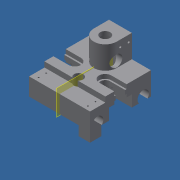
# Autodesk Inventor part: HotendMountCarriage
Saved by Autodesk Inventor 2021 (Build 250183000, 183)
## iProperties
Created: 2022-08-30
Part Number: HotendMountCarriage
Material: Generic
Document SubType Name: Modeling
Designer: Nathann
Density: 1 g/cm^3
Appearance: Default
Author: Nathann
Autodesk Inventor part; units mm, degrees
ref_plane "YZ Plane" through (0, 0, 0) normal (1, 0, 0) x (0, 1, 0)
ref_plane "XZ Plane" through (0, 0, 0) normal (0, 1, 0) x (-1, 0, 0)
ref_plane "XY Plane" through (0, 0, 0) normal (0, 0, 1) x (1, 0, 0)
sketch "Sketch1" plane through (0, 0, 0) normal (0, 0, 1) x (1, 0, 0)
  line L0 (0, 0) -> (80, 0)
  line L1 (80, 0) -> (80, -80)
  line L2 (80, -80) -> (0, -80)
  line L3 (0, -80) -> (0, 0)
  dimension "d0" = 80
  dimension "d1" = 80
  constraints: 8 end point, 2 parallel, 1 horizontal, 1 perpendicular
  measures "d0" distance of L0.start L0.end
  measures "d1" distance of L2.end L0.start
extrude "Extrusion1" add sketch "Sketch1" along normal blind 15
sketch "Sketch2" plane through (0, 0, 0) normal (0, 0, -1) x (-1, 0, 0)
  line L0 (0, 0) -> (-80, 0) projected
  circle A0 centre (-60, -40) radius 6.1
  line L1 (-80, 0) -> (-80, -80) projected
  line L2 (-60, -33.9) -> (-80, -33.9)
  line L3 (-80, -80) -> (-80, 0) projected
  line L4 (-60, -46.1) -> (-80, -46.1)
  line L5 (-80, -46.1) -> (-80, -33.9)
  dimension "d7" = 40
  dimension "d8" = 20
  dimension "d9" = 12.2
  constraints: 6 end point, 2 perpendicular, 2 point on circle, 2 point on line, 1 centre point, 1 horizontal
  measures "d7" distance from line of L0 A0.centre
  measures "d8" distance from line of L1 A0.centre
  measures "d9" diameter of A0
extrude "Extrusion2" cut sketch "Sketch2" against normal through all
sketch "Sketch3" plane through (0, 0, 0) normal (0, 0, -1) x (-1, 0, 0)
  arc A0 (-60, -46.1) -> (-60, -33.9) centre (-60, -40) ccw projected
  circle A1 centre (-60, -40) radius 8.1
  line L0 (-60, -31.9) -> (-80, -31.9)
  line L1 (-80, -33.9) -> (-80, 0) projected
  line L2 (-60, -48.1) -> (-80, -48.1)
  line L3 (-80, -48.1) -> (-80, -31.9)
  point P0 (0, 0)
  dimension "d12" = 16.2
  constraints: 6 end point, 2 horizontal, 2 point on circle, 1 centre point, 1 coincident, 1 perpendicular, 1 point on line
  measures "d12" diameter of A1
extrude "Extrusion3" cut sketch "Sketch3" against normal blind 4
sketch "Sketch4" plane through (0, 0, 15) normal (0, 0, 1) x (1, 0, 0)
  line L0 (80, -31.9) -> (60, -31.9) projected
  arc A0 (60, -31.9) -> (60, -48.1) centre (60, -40) ccw projected
  line L1 (60, -48.1) -> (80, -48.1) projected
  line L2 (80, -46.1) -> (60, -46.1) projected
  arc A1 (60, -33.9) -> (60, -46.1) centre (60, -40) ccw projected
  line L3 (60, -33.9) -> (80, -33.9) projected
  line L4 (80, -33.9) -> (80, -31.9)
  line L5 (80, -33.9) -> (80, 0) projected
  line L6 (80, -46.1) -> (80, -48.1)
  line L7 (80, -80) -> (80, -46.1) projected
  point P0 (0, 0)
  constraints: 4 end point, 2 collinear
extrude "Extrusion4" cut sketch "Sketch4" against normal blind 5.5
sketch "Sketch5" plane through (0, 0, 0) normal (0, 0, -1) x (-1, 0, 0)
  arc A0 (-60, -46.1) -> (-60, -33.9) centre (-60, -40) ccw projected
  line L0 (-80, -31.9) -> (-60, -31.9) projected
  circle A1 centre (-60, -40) radius 8.1
  line L1 (-60, -31.9) -> (-60, -31.9)
  line L2 (-73.8, -31.9) -> (-73.8, -48.1)
  line L3 (-60, -48.1) -> (-60, -48.1)
  arc A2 (-60, -48.1) -> (-60, -31.9) centre (-60, -40) ccw projected
  line L4 (-60, -31.9) -> (-60, -31.9)
  line L5 (-60, -31.9) -> (-60, -31.9)
  line L6 (-60, -33.9) -> (-60, -46.1)
  arc A3 (-60, -31.9) -> (-73.8, -31.9) centre (-66.9, -31.9) ccw
  arc A4 (-73.8, -48.1) -> (-60, -48.1) centre (-66.9, -48.1) ccw
  point P0 (0, 0)
  dimension "d17" = 13.8
  dimension "d20" = 16.2
  dimension "d21" = 8.1
  dimension "d37" = 0
  constraints: 8 end point, 7 point on circle, 4 tangent, 3 centre point, 3 vertical, 1 coincident, 1 parallel, 6 other
  measures "d17" distance of L1.end L2.start
  measures "d20" distance of A4.centre A3.centre
  measures "d21" vertical distance of A1.centre A3.centre
  measures "d37" distance of L0.end L1.end
extrude "Extrusion5" cut sketch "Sketch5" against normal blind 4 contours A3 L0 | L0 A1 A4 L2
sketch "Sketch6" plane through (80, 0, 15) normal (1, 0, 0) x (0, 0, -1)
  line L0 (15, 0) -> (0, 0) projected
  line L1 (15, 0) -> (30, 0)
  line L2 (30, -25) -> (15, -25)
  line L3 (15, -25) -> (15, 0)
  line L4 (15, -80) -> (0, -80) projected
  line L5 (15, -80) -> (30, -80)
  line L6 (30, -55) -> (15, -55)
  line L7 (15, -55) -> (15, -80)
  arc A0 (30, -4.4098) -> (30, -15.5902) centre (25, -10) ccw
  arc A1 (30, -64.4098) -> (30, -75.5902) centre (25, -70) ccw
  line L8 (30, 0) -> (30, -4.4098)
  line L9 (30, -15.5902) -> (30, -25)
  line L10 (30, -80) -> (30, -75.5902)
  line L11 (30, -64.4098) -> (30, -55)
  dimension "d22" = 25
  dimension "d23" = 25
  dimension "d24" = 15
  dimension "d25" = 15
  dimension "d29" = 15
  dimension "d32" = 15
  dimension "d33" = 5
  dimension "d34" = 5
  dimension "d38" = 15
  dimension "d39" = 15
  dimension "d40" = 60
  dimension "d41" = 10
  dimension "d42" = 10
  constraints: 20 end point, 6 parallel, 4 perpendicular, 4 point on circle, 2 centre point, 2 horizontal
  measures "d22" distance of L1.end L2.start
  measures "d23" distance of L5.end L6.start
  measures "d24" distance of L4.start L5.end
  measures "d25" distance of L0.start L1.end
  measures "d29" diameter of A0
  measures "d32" diameter of A1
  measures "d33" distance from line of L8 A0.centre
  measures "d34" distance from line of A1.centre L11
  measures "d38" distance of L2.start L2.end
  measures "d39" distance of L6.start L6.end
  measures "d40" distance of A0.centre A1.centre
  measures "d41" distance from line of L5 A1.centre
  measures "d42" distance from line of L1 A0.centre
extrude "Extrusion6" add sketch "Sketch6" against normal blind 80
ref_plane "Work Plane1" through (40, -33.9, 4) normal (1, 0, 0) x (0, 0, -1)
mirror "Mirror1" about plane through (40, -33.9, 4) normal (1, 0, 0) of "Extrusion5", "Extrusion4", "Extrusion3", "Extrusion2"
sketch "Sketch8" plane through (80, -48.1, 4) normal (1, 0, 0) x (0, 0, -1)
  line L0 (-11, 0) -> (-11, -31.9) projected
  line L1 (-11, -31.9) -> (-4, -31.9)
  line L2 (-4, -31.9) -> (-4, -11.7)
  line L3 (-4, -11.7) -> (-11, -11.7)
  line L4 (-11, -11.7) -> (-11, -31.9)
  point P0 (4, 48.1)
  dimension "d49" = 20.2
  dimension "d50" = 7
  constraints: 8 end point, 2 parallel, 1 horizontal, 1 perpendicular
  measures "d49" distance of L1.end L2.end
  measures "d50" distance of L2.end L3.end
extrude "Extrusion8" cut sketch "Sketch8" along normal through all both and the other way through all
sketch "Sketch9" plane through (80, -80, 8) normal (0, 0, 1) x (1, 0, 0)
  circle A0 centre (-7.6, 14.9) radius 0.95
  circle A1 centre (-7.6, 4.9) radius 0.95
  line L0 (0, 20.2) -> (0, 0) projected
  line L1 (0, 0) -> (-80, 0) projected
  point P0 (-80, 80)
  dimension "d53" = 1.9
  dimension "d54" = 1.9
  dimension "d55" = 7.6
  dimension "d56" = 7.6
  dimension "d57" = 10
  dimension "d58" = 4.9
  constraints: 2 centre point
  measures "d53" diameter of A0
  measures "d54" diameter of A1
  measures "d55" distance from line of A0.centre L0
  measures "d56" distance from line of A1.centre L0
  measures "d57" distance of A1.centre A0.centre
  measures "d58" distance from line of L1 A1.centre
extrude "Extrusion9" cut sketch "Sketch9" against normal blind 10
ref_plane "Work Plane2" through (40, -48.1, 4) normal (1, 0, 0) x (0, 0, -1)
mirror "Mirror2" about plane through (40, -48.1, 4) normal (1, 0, 0) of "Extrusion9"
sketch "Sketch10" plane through (0, 0, 15) normal (0, 0, 1) x (1, 0, 0)
  line L0 (80, -55) -> (0, -55) projected
  circle A0 centre (40, -55) radius 6
  point P0 (0, 0)
  dimension "d61" = 12
  constraints: 1 centre point, 1 midpoint
  measures "d61" diameter of A0
extrude "Extrusion10" cut sketch "Sketch10" against normal through all
sketch "Sketch11" plane through (0, 0, 15) normal (0, 0, 1) x (1, 0, 0)
  circle A0 centre (40, -20) radius 15
  circle A1 centre (40, -20) radius 10
  line L0 (80, -31.9) -> (80, 0) projected
  line L1 (80, 0) -> (0, 0) projected
  line L2 (55, -20) -> (55, -5)
  line L3 (80, -4.4098) -> (0, -4.4098) projected
  line L4 (55, -5) -> (40, -5)
  line L5 (40, -5) -> (25, -5)
  line L6 (25, -5) -> (25, -20)
  line L7 (55, -5) -> (25, -5)
  line L8 (25, -5) -> (25, 0)
  line L9 (25, 0) -> (55, 0)
  line L10 (55, 0) -> (55, -5)
  dimension "d64" = 30
  dimension "d65" = 20
  dimension "d66" = 40
  dimension "d67" = 20
  constraints: 16 end point, 4 perpendicular, 3 point on circle, 2 centre point, 2 parallel, 2 point on line, 1 coincident, 1 horizontal, 1 tangent
  measures "d64" diameter of A0
  measures "d65" diameter of A1
  measures "d66" distance from line of L0 A0.centre
  measures "d67" distance from line of L1 A0.centre
extrude "Extrusion11" add sketch "Sketch11" along normal blind 30 contours A0 | A0 L4 L2 | L5 L8 L3 L10 L4 | A0 L6 L5 | L3 L8 L1 L10
sketch "Sketch12" plane through (0, 0, 45) normal (0, 0, 1) x (1, 0, 0)
  circle A0 centre (40, -20) radius 10 projected
  circle A1 centre (40, -20) radius 6.5
  point P0 (0, 0)
  dimension "d70" = 13
  constraints: 1 centre point, 1 coincident
  measures "d70" diameter of A1
extrude "Extrusion12" add sketch "Sketch12" against normal blind 5
sketch "Sketch13" plane through (0, 0, 15) normal (0, 0, 1) x (1, 0, 0)
  circle A0 centre (40, -20) radius 6.5 projected
  circle A1 centre (40, -20) radius 10
  point P0 (0, 0)
  constraints: 1 centre point, 1 coincident
extrude "Extrusion13" cut sketch "Sketch13" against normal blind 35 contours A0 | A1
sketch "Sketch14" plane through (55, -20, 15) normal (1, 0, 0) x (0, 0, -1)
  circle A0 centre (-21.5, 5) radius 1.45
  circle A1 centre (-21.5, 16) radius 1.45
  line L0 (0, 20) -> (-30, 20) projected
  line L1 (-30, 0) -> (-30, 20) projected
  point P0 (15, 20)
  dimension "d75" = 2.9
  dimension "d76" = 2.9
  dimension "d77" = 11
  dimension "d78" = 4
  dimension "d79" = 8.5
  dimension "d80" = 8.5
  constraints: 2 centre point
  measures "d75" diameter of A0
  measures "d76" diameter of A1
  measures "d77" distance of A1.centre A0.centre
  measures "d78" distance from line of L0 A1.centre
  measures "d79" distance from line of A1.centre L1
  measures "d80" distance from line of A0.centre L1
extrude "Extrusion14" cut sketch "Sketch14" against normal blind 15
sketch "Sketch15" plane through (55, -20, 15) normal (1, 0, 0) x (0, 0, -1)
  circle A0 centre (-8, 0) radius 7.5
  line L0 (15, -10) -> (-25, -10) projected
  line L1 (4, -6) -> (-11, -6)
  line L2 (4, 6) -> (-11, 6)
  line L3 (0, -11.9) -> (0, 20) projected
  point P0 (15, 20)
  dimension "d83" = 6
  dimension "d84" = 15
  dimension "d85" = 8
  constraints: 4 end point, 2 horizontal, 1 centre point, 4 other
  measures "d83" distance from line of A0.centre L2
  measures "d84" diameter of A0
  measures "d85" distance from line of L3 A0.centre
extrude "Extrusion15" cut sketch "Sketch15" against normal blind 17 contours A0
sketch "Sketch16" plane through (0, 0, 0) normal (0, 0, -1) x (-1, 0, 0)
  arc A0 (-34, -55) -> (-46, -55) centre (-40, -55) ccw projected
  arc A1 (-48.6603, -25) -> (-31.3397, -25) centre (-40, -20) ccw projected
  arc A2 (-48.9752, -15.5902) -> (-48.6603, -25) centre (-40, -20) ccw projected
  line L0 (-50, -20) -> (-30, -20)
  line L1 (-30, -20) -> (-30, -55)
  line L2 (-30, -55) -> (-50, -55)
  line L3 (-50, -55) -> (-50, -20)
  arc A3 (-31.3397, -25) -> (-31.0248, -15.5902) centre (-40, -20) ccw projected
  point P0 (0, 0)
  constraints: 8 end point, 2 parallel, 1 horizontal, 1 perpendicular, 1 point on circle, 1 tangent
extrude "Extrusion16" add sketch "Sketch16" along normal blind 15 contours A0 L2 L3 A2 A1 A3 L1
sketch "Sketch17" plane through (80, -25, -15) normal (0, 0, -1) x (-1, 0, 0)
  line L0 (47.5, -22.5) -> (32.5, -22.5)
  line L1 (32.5, -22.5) -> (32.5, -7.5)
  line L2 (32.5, -7.5) -> (47.5, -7.5)
  line L3 (47.5, -7.5) -> (47.5, -22.5)
  line L4 (0, 25) -> (80, 25) projected
  line L5 (80, -6.9) -> (80, 0) projected
  dimension "d90" = 32.5
  dimension "d91" = 15
  dimension "d92" = 15
  dimension "d93" = 32.5
  constraints: 8 end point, 2 parallel, 1 horizontal, 1 perpendicular
  measures "d90" distance between parallel lines of L2 L4
  measures "d91" distance of L2.end L0.start
  measures "d92" distance of L0.start L0.end
  measures "d93" distance between parallel lines of L5 L3
extrude "Extrusion17" add sketch "Sketch17" along normal blind 45
sketch "Sketch18" plane through (32.5, -32.5, -15) normal (0, 1, 0) x (1, 0, 0)
  circle A0 centre (7.5, 37.5) radius 7.5
  line L0 (0, 45) -> (15, 45) projected
  line L1 (0, 0) -> (0, 45) projected
  point P0 (-32.5, -15)
  dimension "d96" = 7.5
  dimension "d97" = 7.5
  dimension "d98" = 15
  constraints: 1 centre point
  measures "d96" distance from line of L0 A0.centre
  measures "d97" distance from line of L1 A0.centre
  measures "d98" diameter of A0
extrude "Extrusion18" add sketch "Sketch18" along normal blind 32.5 contours A0
ref_plane "Work Plane3" through (40, -5, -52.5) normal (0, 1, 0) x (1, 0, 0)
sketch "Sketch19" plane through (40, -5, -52.5) normal (0, 1, 0) x (1, 0, 0)
  arc A0 (7.5, 0) -> (0, 7.5) centre (0, 0) ccw projected
  circle A1 centre (0, 0) radius 7.5
  circle A2 centre (0, 0) radius 5
  point P0 (-40, -52.5)
  dimension "d102" = 10
  constraints: 2 coincident, 1 centre point, 3 other
  measures "d102" diameter of A2
extrude "Extrusion19" cut sketch "Sketch19" against normal blind 5
sketch "Sketch20" plane through (80, -25, -60) normal (0, 0, -1) x (-1, 0, 0)
  line L0 (32.5, -22.5) -> (32.5, -7.5) projected
  arc A0 (33.2483, -18.2) -> (34, -19.5) centre (32.5, -19.5) ccw
  line L1 (32.5, -22.5) -> (47.5, -22.5) projected
  circle A1 centre (35.5, -19.5) radius 1.5
  circle A2 centre (41.5, -19.5) radius 1.5
  circle A3 centre (47.5, -19.5) radius 1.5
  arc A4 (45.2483, -20.8) -> (44.9, -19.5) centre (47.5, -19.5) ccw
  circle A5 centre (44.5, -19.5) radius 0.4
  circle A6 centre (38.5, -19.5) radius 0.4
  circle A7 centre (32.5, -19.5) radius 0.4
  arc A8 (45.1708, -18.3446) -> (43.8292, -18.3446) centre (44.5, -19.5) ccw
  arc A9 (43, -19.5) -> (46, -19.5) centre (44.5, -19.5) ccw
  arc A10 (44.1, -19.5) -> (38.9, -19.5) centre (41.5, -19.5) ccw
  arc A11 (39.7083, -20.3888) -> (43.2917, -20.3888) centre (41.5, -19.5) ccw
  arc A12 (39.1708, -18.3446) -> (37.8292, -18.3446) centre (38.5, -19.5) ccw
  arc A13 (37, -19.5) -> (40, -19.5) centre (38.5, -19.5) ccw
  arc A14 (38.1, -19.5) -> (32.9, -19.5) centre (35.5, -19.5) ccw
  arc A15 (33.7083, -20.3888) -> (37.2917, -20.3888) centre (35.5, -19.5) ccw
  line L2 (47.5, -16.9) -> (47.5, -22.1)
  line L3 (32.5, -18) -> (32.5, -21)
  line L4 (47.5, -15) -> (32.5, -15)
  arc A16 (34, -10.5) -> (33.2483, -11.8) centre (32.5, -10.5) ccw
  line L5 (32.5, -7.5) -> (47.5, -7.5)
  circle A17 centre (35.5, -10.5) radius 1.5
  circle A18 centre (41.5, -10.5) radius 1.5
  circle A19 centre (47.5, -10.5) radius 1.5
  arc A20 (44.9, -10.5) -> (45.2483, -9.2) centre (47.5, -10.5) ccw
  circle A21 centre (44.5, -10.5) radius 0.4
  circle A22 centre (38.5, -10.5) radius 0.4
  circle A23 centre (32.5, -10.5) radius 0.4
  arc A24 (43.8292, -11.6554) -> (45.1708, -11.6554) centre (44.5, -10.5) ccw
  arc A25 (46, -10.5) -> (43, -10.5) centre (44.5, -10.5) ccw
  arc A26 (38.9, -10.5) -> (44.1, -10.5) centre (41.5, -10.5) ccw
  arc A27 (43.2917, -9.6112) -> (39.7083, -9.6112) centre (41.5, -10.5) ccw
  arc A28 (37.8292, -11.6554) -> (39.1708, -11.6554) centre (38.5, -10.5) ccw
  arc A29 (40, -10.5) -> (37, -10.5) centre (38.5, -10.5) ccw
  arc A30 (32.9, -10.5) -> (38.1, -10.5) centre (35.5, -10.5) ccw
  arc A31 (37.2917, -9.6112) -> (33.7083, -9.6112) centre (35.5, -10.5) ccw
  line L6 (47.5, -13.1) -> (47.5, -7.9)
  line L7 (32.5, -12) -> (32.5, -9)
  point P0 (80, 25)
  point P1 (47.5, -18)
  point P2 (32.5, -19.9)
  point P3 (47.5, -12)
  point P4 (32.5, -9)
  point P5 (32.5, -10.1)
  dimension "d120" = 3
  dimension "d114" = 3
  dimension "d115" = 3
  dimension "d116" = 3
  dimension "d118" = 3
  dimension "d121" = 5.2
  dimension "d122" = 7.5
  constraints: 84 point on circle, 37 symmetric about line, 28 centre point, 12 coincident, 12 end point, 4 point on line, 2 horizontal, 2 tangent, 1 midpoint, 1 perpendicular, 1 vertical, 26 other
  measures "d114" diameter of A0
  measures "d115" distance from line of L1 A0.centre
  measures "d116" diameter of A1
  measures "d118" diameter of A2
  measures "d121" diameter of A4
  measures "d122" distance between parallel lines of L1 L4
extrude "Extrusion20" cut sketch "Sketch20" against normal blind 20 contours L0 A7 A14 A6 A10 A5 A4 L2 A3 A9 A2 A13 A1 A0 | A16 A17 A29 A18 A25 A19 L6 A20 A21 A26 A22 A30 A23 L0
equation "\"d24\" = d25"
equation "\"d32\" = d29"
equation "\"d34\" = d33"
equation "\"d75\" = d76"
equation "\"d80\" = d79"
equation "\"d93\" = d90"
equation "\"d97\" = d96"
equation "\"d118\" = d117"
equation "\"RodDiameter\" = 8"
equation "\"VerticalBearingOD\" = 16"
equation "\"PrintingClearance\" = 0.2"
equation "\"d31\" = d30"
equation "\"TubeID\" = 18"
equation "\"d117\" = 3"
equation "\"d30\" = 5"
body "Solid1"
